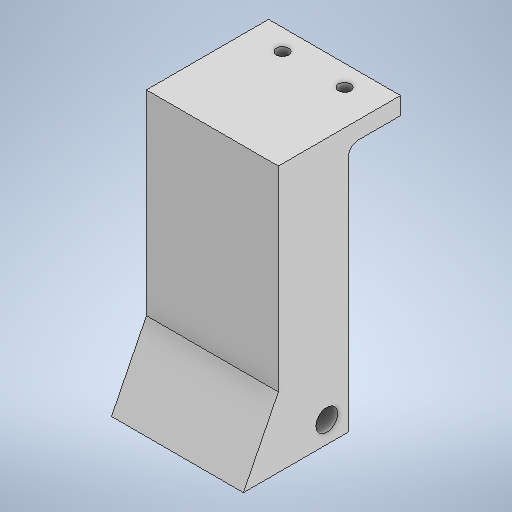
# Autodesk Inventor part: legsv1
Saved by Autodesk Inventor 2025.2 (Build 292293000, 293)
## iProperties
Created: 2025-04-24
Part Number: legsv1
Material: Generic
Document SubType Name: Modeling
Designer: patrickandersen
Density: 1 g/cm^3
Appearance: Default
Author: patrickandersen
Autodesk Inventor part; units mm, degrees
ref_plane "YZ Plane" through (0, 0, 0) normal (1, 0, 0) x (0, 1, 0)
ref_plane "XZ Plane" through (0, 0, 0) normal (0, 1, 0) x (-1, 0, 0)
ref_plane "XY Plane" through (0, 0, 0) normal (0, 0, 1) x (1, 0, 0)
sketch "Sketch1" plane through (0, 0, 0) normal (0, 1, 0) x (-1, 0, 0)
  line L0 (16.9826, -9.4) -> (-20.8174, -9.4)
  line L1 (-20.8174, -9.4) -> (-20.8174, -29.4)
  line L2 (-20.8174, -29.4) -> (16.9826, -29.4)
  line L3 (16.9826, -29.4) -> (16.9826, -9.4)
  line L4 (7.0826, -29.4) -> (-10.9174, -29.4)
  line L5 (-10.9174, -29.4) -> (-10.9174, -17.15)
  line L6 (-10.9174, -17.15) -> (7.0826, -17.15)
  line L7 (7.0826, -17.15) -> (7.0826, -29.4)
  point P0 (0, 0)
  dimension "d0" = 37.8
  dimension "d1" = 20
  dimension "d2" = 9.9
  dimension "d3" = 9.9
  dimension "d4" = 12.25
  constraints: 16 end point, 4 parallel, 2 horizontal, 2 perpendicular, 1 point on line
  measures "d0" distance of L1.end L2.end
  measures "d1" distance of L2.end L0.start
  measures "d2" distance between parallel lines of L3 L7
  measures "d3" distance between parallel lines of L1 L5
  measures "d4" distance of L6.end L4.start
extrude "Extrusion1" add sketch "Sketch1" along normal blind 76.05
extrude "Extrusion2" cut sketch "Sketch1" along normal blind 12.25 contours L2 L5 L6 L7
sketch "Sketch2" plane through (0, 0, 0) normal (0, -1, 0) x (1, 0, 0)
  line L0 (-16.9826, -29.4) -> (-16.9826, -9.4) projected
  line L1 (-16.9826, -9.4) -> (20.8174, -9.4)
  line L2 (20.8174, -9.4) -> (20.8174, 0.6)
  line L3 (20.8174, 0.6) -> (-16.9826, 0.6)
  line L4 (-16.9826, 0.6) -> (-16.9826, -9.4)
  point P0 (0, 0)
  dimension "d10" = 10
  constraints: 8 end point, 2 parallel, 1 horizontal, 1 perpendicular
  measures "d10" distance of L3.end L0.end
extrude "Extrusion3" add sketch "Sketch2" against normal blind 20
sketch "Sketch4" plane through (20.8174, 0, -29.4) normal (1, 0, 0) x (0, 0, -1)
  line L0 (0, 0) -> (-30, 0) projected
  line L1 (-30, 0) -> (-30, 20) projected
  line L2 (-30, 0) -> (-30, 20)
  line L3 (-30, 20) -> (-20, 20)
  line L4 (-30, 0) -> (-30, 20)
  line L5 (-20, 20) -> (-30, 0)
  point P0 (-29.4, 0)
  dimension "d14" = 10
  constraints: 8 end point, 2 collinear, 1 perpendicular
  measures "d14" distance of L1.end L3.end
extrude "Extrusion4" cut sketch "Sketch4" against normal blind 50
sketch "Sketch5" plane through (20.8174, 76.05, -29.4) normal (0, 0, -1) x (-1, 0, 0)
  line L0 (0, -76.05) -> (0, 0) projected
  line L1 (37.8, 0) -> (0, 0)
  line L2 (0, 0) -> (0, -5)
  line L3 (0, -5) -> (37.8, -5)
  line L4 (37.8, -5) -> (37.8, 0)
  point P0 (20.8174, -76.05)
  dimension "d17" = 5
  constraints: 8 end point, 2 parallel, 1 horizontal, 1 perpendicular, 1 point on line
  measures "d17" distance of L3.end L1.start
extrude "Extrusion5" add sketch "Sketch5" along normal blind 15
fillet "Fillet2" radius 3 1 edges at (1.9174, 71.05, -29.4)
sketch "Sketch6" plane through (-16.9826, 0, -29.4) normal (-1, 0, 0) x (0, 0, 1)
  circle A0 centre (6.125, 6.125) radius 3.125
  line L0 (0, 0) -> (30, 0) projected
  line L1 (0, 0) -> (0, 68.05) projected
  point P0 (29.4, 0)
  dimension "d21" = 6.25
  dimension "d22" = 6.125
  dimension "d23" = 6.125
  constraints: 1 centre point
  measures "d21" diameter of A0
  measures "d22" distance from line of L0 A0.centre
  measures "d23" distance from line of L1 A0.centre
hole "Hole1" at (-16.9826, 6.125, -23.275) direction (1, 0, 0) diameter 6.25 end through all
sketch "Sketch7" plane through (-16.9826, 71.05, -44.4) normal (0, -1, 0) x (1, 0, 0)
  circle A0 centre (10, 6) radius 2.75
  circle A1 centre (27.8, 6) radius 2.75
  line L0 (0, 12) -> (0, 0) projected
  line L1 (37.8, 12) -> (37.8, 0) projected
  line L2 (37.8, 0) -> (0, 0) projected
  line L3 (0, 12) -> (37.8, 12) projected
  point P0 (16.9826, 44.4)
  point P1 (37.8, 6)
  dimension "d32" = 5.5
  dimension "d33" = 5.5
  dimension "d34" = 10
  dimension "d35" = 10
  dimension "d36" = 6
  dimension "d37" = 6
  dimension "d38" = 6
  constraints: 2 centre point, 1 midpoint
  measures "d32" diameter of A0
  measures "d33" diameter of A1
  measures "d34" distance from line of L0 A0.centre
  measures "d35" distance of point (37.8, 6) A1.centre
  measures "d36" distance from line of L2 A0.centre
  measures "d37" distance from line of L3 A0.centre
  measures "d38" distance from line of L2 A1.centre
hole "Hole2" at (-6.9826, 71.05, -38.4) at (10.8174, 71.05, -38.4) direction (0, 1, 0) diameter 3.5 end through all
body "Solid1"
